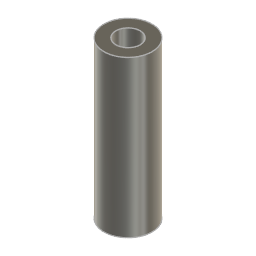
link piece right (Autodesk Fusion 360 design; units mm, degrees)
Autodesk Fusion 360 part; units mm, degrees
sketch "Sketch1" plane through (0, 0, 0) normal (0, 0, 1) x (1, 0, 0)
  line L0 (1.8764, -3.25) -> (3.7528, 0)
  line L1 (3.7528, 0) -> (1.8764, 3.25)
  line L2 (1.8764, 3.25) -> (-1.8764, 3.25)
  line L3 (-1.8764, 3.25) -> (-3.7528, 0)
  line L4 (-3.7528, 0) -> (-1.8764, -3.25)
  line L5 (-1.8764, -3.25) -> (1.8764, -3.25)
  circle A0 centre (0, 0) radius 4.75
  dimension "d1" = 3.25
  dimension "d2" = 9.5
  constraint coincident A0.centre origin
  constraint horizontal L5
  measures "d1" distance of A0.centre L5
  measures "d2" diameter of A0
extrude "Extrude1" add sketch "Sketch1" along normal blind 13
sketch "Sketch2" plane through (0, 0, 13) normal (0, 0, 1) x (-1, 0, 0)
  line L0 (-1.8764, 3.25) -> (1.8764, 3.25)
  line L1 (1.8764, 3.25) -> (3.7528, 0)
  line L2 (3.7528, 0) -> (1.8764, -3.25)
  line L3 (1.8764, -3.25) -> (-1.8764, -3.25)
  line L4 (-1.8764, -3.25) -> (-3.7528, 0)
  line L5 (-3.7528, 0) -> (-1.8764, 3.25)
  circle A0 centre (0, 0) radius 4.75
extrude "Extrude2" add sketch "Sketch2" along normal blind 1 contours L0 L1 L2 L3 L4 L5 | A0
sketch "Sketch3" plane through (0, 0, 14) normal (0, 0, 1) x (-1, 0, 0)
  circle A0 centre (0, 0) radius 4.75
  circle A1 centre (0, 0) radius 2.4
  dimension "d7" = 4.8
  constraint coincident A0.centre A1.centre
  measures "d7" diameter of A1
extrude "Extrude3" add sketch "Sketch3" along normal blind 16.8
named bodies: "link right"
